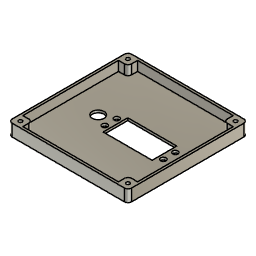
TRARM02_Base_Top_100x100x10 (Autodesk Fusion 360 design; units mm, degrees)
Autodesk Fusion 360 part; units mm, degrees
sketch "스케치1" plane through (0, 0, 0) normal (0, 0, 1) x (1, 0, 0)
  line L0 (0, 0) -> (100, 0)
  line L1 (100, 0) -> (100, 100)
  line L2 (100, 100) -> (0, 100)
  line L3 (0, 100) -> (0, 0)
  dimension "d1" = 100
  dimension "d2" = 100
  constraint horizontal L0
  constraint vertical L1
  constraint horizontal L2
  constraint vertical L3
  constraint coincident L0.start L3.end
  measures "d1" distance of L0.start L0.end
  measures "d2" distance of L0.start L2.end
extrude "돌출1" add sketch "스케치1" along normal blind 2
sketch "스케치2" plane through (0, 0, 2) normal (0, 0, 1) x (-1, 0, 0)
  line L0 (0, -100) -> (-100, -100)
  line L1 (-100, -100) -> (-100, 0)
  line L2 (-100, 0) -> (0, 0)
  line L3 (0, 0) -> (0, -100)
  line L4 (-10, -98) -> (-90, -98)
  line L5 (-98, -90) -> (-98, -10)
  line L6 (-90, -2) -> (-10, -2)
  line L7 (-2, -10) -> (-2, -90)
  line L8 (-2, -90) -> (-10, -90)
  line L9 (-10, -90) -> (-10, -98)
  line L10 (-90, -98) -> (-90, -90)
  line L11 (-90, -90) -> (-98, -90)
  line L12 (-98, -10) -> (-90, -10)
  line L13 (-90, -10) -> (-90, -2)
  line L14 (-10, -2) -> (-10, -10)
  line L15 (-10, -10) -> (-2, -10)
  point P0 (0, -100)
  point P1 (-100, 0)
  dimension "d5" = 2
  dimension "d6" = 2
  dimension "d7" = 8
  dimension "d8" = 8
  dimension "d9" = 2
  dimension "d10" = 2
  dimension "d11" = 8
  dimension "d12" = 8
  constraint horizontal L0
  constraint vertical L1
  constraint horizontal L2
  constraint vertical L3
  constraint coincident P1 L1.end
  constraint coincident P0 L0.start
  constraint horizontal L4
  constraint vertical L5
  constraint horizontal L6
  constraint vertical L7
  constraint perpendicular L7 L8
  constraint perpendicular L4 L9
  constraint perpendicular L4 L10
  constraint perpendicular L5 L11
  constraint perpendicular L5 L12
  constraint perpendicular L6 L13
  constraint perpendicular L6 L14
  constraint perpendicular L7 L15
  constraint equal L11 L12
  constraint equal L9 L14
  constraint equal L13 L14
  constraint equal L8 L11
  measures "d5" distance of L3 L7
  measures "d6" distance of L2 L6
  measures "d7" distance of L14.end L7.start
  measures "d8" distance of L6.end L14.end
  measures "d9" distance of L1 L5
  measures "d10" distance of L0 L4
  measures "d11" distance of L10.end L5.start
  measures "d12" distance of L4.end L10.end
extrude "돌출2" add sketch "스케치2" along normal blind 8
sketch "스케치3" plane through (0, 0, 10) normal (0, 0, 1) x (-1, 0, 0)
  circle A0 centre (-5, -95) radius 1.5
  circle A1 centre (-95, -95) radius 1.5
  circle A2 centre (-95, -5) radius 1.5
  circle A3 centre (-5, -5) radius 1.5
  dimension "d15" = 3
  dimension "d16" = 5
  dimension "d17" = 5
  dimension "d18" = 90
  dimension "d19" = 90
  constraint equal A2 A3
  constraint equal A0 A1
  constraint equal A1 A2
  constraint horizontal A2.centre A3.centre
  constraint vertical A1.centre A2.centre
  constraint vertical A0.centre A3.centre
  constraint horizontal A0.centre A1.centre
  measures "d15" diameter of A0
  measures "d16" horizontal distance of origin A3.centre
  measures "d17" vertical distance of origin A3.centre
  measures "d18" distance of A2.centre A3.centre
  measures "d19" distance of A0.centre A3.centre
extrude "돌출3" cut sketch "스케치3" against normal blind 10
fillet "필렛1" radius 3 4 edges at (0, 0, 5) (100, 0, 5) (100, 100, 5) (0, 100, 5)
fillet "필렛1" radius 3 4 edges at (10, 90, 6) (10, 10, 6) (90, 90, 6) (90, 10, 6)
chamfer "챔퍼1" distance 2 angle 45 4 edges at (6.3985, 95.5424, 0) (6.3985, 5.5424, 0) (96.3985, 5.5424, 0) (96.3985, 95.5424, 0)
sketch "스케치4" plane through (0, 0, 2) normal (0, 0, 1) x (-1, 0, 0)
  line L0 (-39.5, -60.3) -> (-80.5, -60.3)
  line L1 (-80.5, -60.3) -> (-80.5, -39.7)
  line L2 (-80.5, -39.7) -> (-39.5, -39.7)
  line L3 (-39.5, -39.7) -> (-39.5, -60.3)
  circle A0 centre (-35.5, -55.1) radius 2.25
  circle A1 centre (-35.5, -45.1) radius 2.25
  circle A2 centre (-84.5, -55.1) radius 2.25
  circle A3 centre (-84.5, -45.1) radius 2.25
  circle A4 centre (-25, -50) radius 5
  point P0 (-3, -100)
  dimension "d27" = 20.6
  dimension "d28" = 41
  dimension "d29" = 39.5
  dimension "d33" = 10
  dimension "d34" = 49
  dimension "d35" = 4.5
  dimension "d37" = 5.4
  dimension "d41" = 39.7
  dimension "d43" = 4
  dimension "d45" = 10
  dimension "d46" = 25
  dimension "d47" = 50
  constraint horizontal L0
  constraint vertical L1
  constraint horizontal L2
  constraint vertical L3
  constraint equal A2 A3
  constraint equal A0 A2
  constraint equal A0 A1
  constraint horizontal A0.centre A2.centre
  constraint vertical A0.centre A1.centre
  constraint horizontal A1.centre A3.centre
  constraint vertical A2.centre A3.centre
  measures "d27" distance of L0.end L1.end
  measures "d28" distance of L1.end L2.end
  measures "d29" horizontal distance of origin L2.end
  measures "d33" distance of A0.centre A1.centre
  measures "d34" distance of A0.centre A2.centre
  measures "d35" diameter of A2
  measures "d37" vertical distance of L2.end A1.centre
  measures "d41" vertical distance of origin L2.end
  measures "d43" horizontal distance of L2.end A1.centre
  measures "d45" diameter of A4
  measures "d46" horizontal distance of origin A4.centre
  measures "d47" vertical distance of origin A4.centre
extrude "돌출4" cut sketch "스케치4" against normal blind 2
